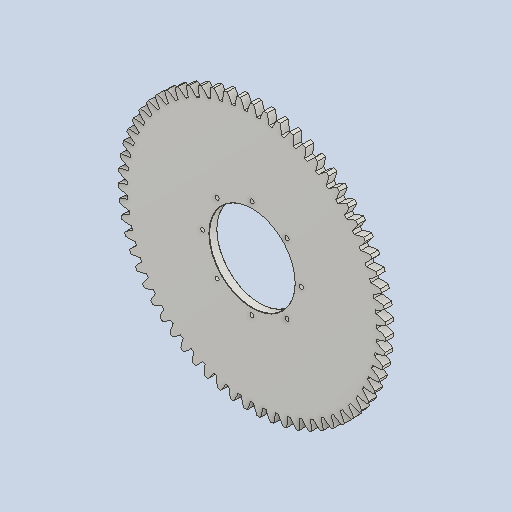
# Autodesk Inventor part: ДМФ 01 41 Шестерня ведомая
Saved by Autodesk Inventor 2024.2 (Build 282272000, 272)
## iProperties
CustomPartVersion: 1
Created: 2024-04-25
Part Number: ДМФ 01 41 Шестерня ведомая
Material: Steel
Document SubType Name: Modeling
Designer: pokla
Categories: <?xml version="1.0" encoding="UTF-16"?> <MemberInstance><Categories><FamilyTemplate><FamilyTemplateParameter ValueType="xs:double" Id="1" ObjectReferenceKey="da_z" ObjectType="kUserParameterObject"/><FamilyTemplateParameter ValueType="xs:double" Id="2" ObjectReferenceKey="da_b" ObjectType="kUserParameterObject"/><FamilyTemplateParameter ValueType="xs:double" Id="3" ObjectReferenceKey="da_beta" ObjectType="kUserParameterObject"/><FamilyTemplateParameter ValueType="xs:double" Id="4" ObjectReferenceKey="da_da" ObjectType="kUserParameterObject"/><FamilyTemplateParameter ValueType="xs:double" Id="5" ObjectReferenceKey="da_aw" ObjectType="kUserParameterObject"/><FamilyTemplateParameter ValueType="xs:string" Id="6" ObjectReferenceKey="EAIAABAAAACIAQAAAAAAAIAAAAAAAAAA" ObjectType="83910656" SubObjectId="SurfaceGeometry"/></FamilyTemplate><ParamToTemplateMap><ParamToTemplate CategoryParameter="//CategoryParameter[@InternalName='046C89C9-8512-4d59-83FE-43B91F4F132A']" TemplateParameter="1"/><ParamToTemplate CategoryParameter="//CategoryParameter[@InternalName='2552DF32-E462-4b46-AEBF-C6C7768E72AC']" TemplateParameter="2"/><ParamToTemplate CategoryParameter="//CategoryParameter[@InternalName='C9EE641D-15FC-4fae-A226-E94C4372FDD7']" TemplateParameter="3"/><ParamToTemplate><ParamToTemplate CategoryParameter="//CategoryParameter[@InternalName='00B6519A-459B-49c7-AD84-2E56D39A5744']" ConstantValue="0.000029"/></ParamToTemplate><ParamToTemplate><ParamToTemplate CategoryParameter="//CategoryParameter[@InternalName='04B31F0E-C7A6-4894-AA32-9629BEFACF47']" ConstantValue="1.000000"/></ParamToTemplate><ParamToTemplate><ParamToTemplate CategoryParameter="//CategoryParameter[@InternalName='43CBEC2E-7847-49e7-A936-2F7889FCB2D9']" ConstantValue="0.250000"/></ParamToTemplate><ParamToTemplate><ParamToTemplate CategoryParameter="//CategoryParameter[@InternalName='B1EFC894-105D-4ebd-86BF-FA20ED196853']" ConstantValue="0.333500"/></ParamToTemplate><ParamToTemplate><ParamToTemplate CategoryParameter="//CategoryParameter[@InternalName='51175063-3D10-4879-93E8-6246FE8B403D']" ConstantValue="2060000000.000000"/></ParamToTemplate><ParamToTemplate><ParamToTemplate CategoryParameter="//CategoryParameter[@InternalName='A3A52E27-4454-46a9-B0BD-C932399B70AF']" ConstantValue="0.300000"/></ParamToTemplate><ParamToTemplate><ParamToTemplate CategoryParameter="//CategoryParameter[@InternalName='91B76062-C214-41d9-B1B9-14D2AB99603D']" ConstantValue="1.250632"/></ParamToTemplate><ParamToTemplate><ParamToTemplate CategoryParameter="//CategoryParameter[@InternalName='374E806E-8B8A-4dda-A9AA-1039D6500AD2']" ConstantValue="0.799596"/></ParamToTemplate><ParamToTemplate><ParamToTemplate CategoryParameter="//CategoryParameter[@InternalName='2D373A89-B862-43d6-8D0B-0CBF12AB9F6C']" ConstantValue="0.253073"/></ParamToTemplate><ParamToTemplate CategoryParameter="//CategoryParameter[@InternalName='37777632-D6A2-4fac-9D53-DB8ACD95C989']" TemplateParameter="4"/><ParamToTemplate CategoryParameter="//CategoryParameter[@InternalName='FD1017F1-B727-4f7e-9707-0F86F1FF9423']" TemplateParameter="5"/><ParamToTemplate><ParamToTemplate CategoryParameter="//CategoryParameter[@InternalName='9E1B4470-B2D3-4ff1-B813-535BB4CDF51A']" ConstantValue="3520000.000000"/></ParamToTemplate><ParamToTemplate><ParamToTemplate CategoryParameter="//CategoryParameter[@InternalName='F8452263-BFF6-458c-9FB1-07C4B99E95CD']" ConstantValue="11400000.000000"/></ParamToTemplate><ParamToTemplate><ParamToTemplate CategoryParameter="//CategoryParameter[@InternalName='3E3BB259-FD49-497f-8171-6EBC954A3479']" ConstantValue="2.000000"/></ParamToTemplate><ParamToTemplate CategoryParameter="//CategoryParameter[@InternalName='27C3BAF2-7550-4e4b-AE2C-0DB134B7D9B7']" TemplateParameter="6"/></ParamToTemplateMap><Category DisplayName="Gear" InternalName="DC85795E-93AB-48d5-8EEE-5A27447B64BD" Mnemonic="Gear"><CategoryParameter DisplayName="z" InternalName="046C89C9-8512-4d59-83FE-43B91F4F132A" Mnemonic="z"/><CategoryParameter DisplayName="b" InternalName="2552DF32-E462-4b46-AEBF-C6C7768E72AC" Mnemonic="b"/><CategoryParameter DisplayName="||b|" InternalName="C9EE641D-15FC-4fae-A226-E94C4372FDD7" Mnemonic="beta"/><CategoryParameter DisplayName="x" InternalName="00B6519A-459B-49c7-AD84-2E56D39A5744" Mnemonic="x"/><CategoryParameter DisplayName="a*" InternalName="04B31F0E-C7A6-4894-AA32-9629BEFACF47" Mnemonic="a"/><CategoryParameter DisplayName="c*" InternalName="43CBEC2E-7847-49e7-A936-2F7889FCB2D9" Mnemonic="c"/><CategoryParameter DisplayName="r|.f|*" InternalName="B1EFC894-105D-4ebd-86BF-FA20ED196853" Mnemonic="rf"/><CategoryParameter DisplayName="E" InternalName="51175063-3D10-4879-93E8-6246FE8B403D" Mnemonic="E"/><CategoryParameter DisplayName="||m|" InternalName="A3A52E27-4454-46a9-B0BD-C932399B70AF" Mnemonic="mi"/><Category DisplayName="SpurGear" InternalName="26C5A22E-A91E-4dfd-A3B3-23CCAFAE1764" Mnemonic="SpurGear"><CategoryParameter DisplayName="m" InternalName="91B76062-C214-41d9-B1B9-14D2AB99603D" Mnemonic="m"/><CategoryParameter DisplayName="P" InternalName="374E806E-8B8A-4dda-A9AA-1039D6500AD2" Mnemonic="PP"/><CategoryParameter DisplayName="||a|" InternalName="2D373A89-B862-43d6-8D0B-0CBF12AB9F6C" Mnemonic="alpha"/><CategoryParameter DisplayName="d|.a|" InternalName="37777632-D6A2-4fac-9D53-DB8ACD95C989" Mnemonic="da"/><CategoryParameter DisplayName="a|.w|" InternalName="FD1017F1-B727-4f7e-9707-0F86F1FF9423" Mnemonic="aw"/><CategoryParameter DisplayName="||s||.Flim|" InternalName="9E1B4470-B2D3-4ff1-B813-535BB4CDF51A" Mnemonic="sFlim"/><CategoryParameter DisplayName="||s||.Hlim|" InternalName="F8452263-BFF6-458c-9FB1-07C4B99E95CD" Mnemonic="sHlim"/><CategoryParameter DisplayName="type" InternalName="3E3BB259-FD49-497f-8171-6EBC954A3479" Mnemonic="type"/><CategoryParameter DisplayName="PitchDiameter" InternalName="27C3BAF2-7550-4e4b-AE2C-0DB134B7D9B7" Mnemonic="IDS_PITCHDIAM"/></Category></Category></Categories></MemberInstance>
Density: 1 g/cm^3
Appearance: Steel
Author: pokla
Autodesk Inventor part; units mm, degrees
ref_plane "YZ Plane" through (0, 0, 0) normal (1, 0, 0) x (0, 1, 0)
ref_plane "XZ Plane" through (0, 0, 0) normal (0, 1, 0) x (-1, 0, 0)
ref_plane "XY Plane" through (0, 0, 0) normal (0, 0, 1) x (1, 0, 0)
sketch "Sketch1" plane through (0, 0, 0) normal (0, 0, 1) x (1, 0, 0)
  circle A0 centre (0, 0) radius 406.4558
  dimension "d0" = 812.9115
  constraints: 1 centre point
  measures "d0" diameter of A0
extrude "Extrusion1" add sketch "Sketch1" along normal blind 24
ref_plane "Work Plane2" through (0, 0, 12) normal (0, 0, 1) x (1, 0, 0)
sketch "Sketch2" plane through (0, 0, 0) normal (0, 0, -1) x (-1, 0, 0)
  circle A0 centre (0, 0) radius 406.4558 projected
  circle A1 centre (0, 0) radius 393.9491
  dimension "d3" = 787.8982
  constraints: 1 centre point, 1 coincident
  measures "d3" diameter of A1
surface extrude "Pitch Diameter" sketch "Sketch2" against normal through all shown no curves A1
ref_plane "Work Plane8" through (0, 0, 0) normal (0.9987569, 0.0498459, 0) x (0, 0, 1)
ref_plane "Work Plane9" through (0, 0, 0) normal (1, 0, 0) x (0, 1, 0)
spur gear teeth "Spur Gear" teeth 63 pitch diameter 787.8982 tip diameter 812.9115 root diameter 756.6331 face width 24 start plane through (0, 0, 0) normal (0, 0, -1) x (-1, 0, 0)
sketch "Sketch3" plane through (0, 0, 24) normal (0, 0, 1) x (1, 0, 0)
  arc A0 (-35.425, 404.9091) -> (-45.5086, 403.9001) centre (0, 0) ccw projected
  arc A1 (-45.5086, 403.9001) -> (-51.7172, 374.7649) centre (107.0022, 356.1713) ccw projected
  arc A2 (-51.7172, 374.7649) -> (-61.0443, 373.3591) centre (0, 0) ccw projected
  arc A3 (-61.0443, 373.3591) -> (-75.5648, 399.3698) centre (-207.2317, 308.8081) ccw projected
  arc A4 (-75.5648, 399.3698) -> (-85.4979, 397.3618) centre (0, 0) ccw projected
  arc A5 (-85.4979, 397.3618) -> (-88.7748, 367.7532) centre (71.0072, 365.0554) ccw projected
  arc A6 (-88.7748, 367.7532) -> (-97.9155, 365.4257) centre (0, 0) ccw projected
  arc A7 (-97.9155, 365.4257) -> (-114.9537, 389.8614) centre (-236.9493, 286.64) ccw projected
  arc A8 (-114.9537, 389.8614) -> (-124.6375, 386.8744) centre (0, 0) ccw projected
  arc A9 (-124.6375, 386.8744) -> (-124.95, 357.0867) centre (34.3066, 370.3114) ccw projected
  arc A10 (-124.95, 357.0867) -> (-133.8136, 353.8606) centre (0, 0) ccw projected
  arc A11 (-133.8136, 353.8606) -> (-153.2002, 376.4784) centre (-264.3119, 261.6231) ccw projected
  arc A12 (-153.2002, 376.4784) -> (-162.5384, 372.542) centre (0, 0) ccw projected
  arc A13 (-162.5384, 372.542) -> (-159.8835, 342.8712) centre (-2.735, 371.887) ccw projected
  arc A14 (-159.8835, 342.8712) -> (-168.3818, 338.7786) centre (0, 0) ccw projected
  arc A15 (-168.3818, 338.7786) -> (-189.924, 359.3538) centre (-289.0478, 234.0061) ccw projected
  arc A16 (-189.924, 359.3538) -> (-198.8239, 354.5072) centre (0, 0) ccw projected
  arc A17 (-198.8239, 354.5072) -> (-193.2279, 325.2482) centre (-39.7494, 369.7667) ccw projected
  arc A18 (-193.2279, 325.2482) -> (-201.2765, 320.3298) centre (0, 0) ccw projected
  arc A19 (-201.2765, 320.3298) -> (-224.7603, 338.6578) centre (-310.9109, 204.0634) ccw projected
  arc A20 (-224.7603, 338.6578) -> (-233.1334, 332.9491) centre (0, 0) ccw projected
  arc A21 (-233.1334, 332.9491) -> (-224.652, 304.3926) centre (-76.3687, 363.9715) ccw projected
  arc A22 (-224.652, 304.3926) -> (-232.1709, 298.6973) centre (0, 0) ccw projected
  arc A23 (-232.1709, 298.6973) -> (-257.3629, 314.596) centre (-329.6841, 172.0926) ccw projected
  arc A24 (-257.3629, 314.596) -> (-265.126, 308.082) centre (0, 0) ccw projected
  arc A25 (-265.126, 308.082) -> (-253.8434, 280.5119) centre (-112.2291, 354.559) ccw projected
  arc A26 (-253.8434, 280.5119) -> (-260.7578, 274.0963) centre (0, 0) ccw projected
  arc A27 (-260.7578, 274.0963) -> (-287.4076, 287.4076) centre (-345.1807, 138.4115) ccw projected
  arc A28 (-287.4076, 287.4076) -> (-294.4836, 280.153) centre (0, 0) ccw projected
  arc A29 (-294.4836, 280.153) -> (-280.5119, 253.8434) centre (-146.9741, 341.6227) ccw projected
  arc A30 (-280.5119, 253.8434) -> (-286.7532, 246.7711) centre (0, 0) ccw projected
  arc A31 (-286.7532, 246.7711) -> (-314.596, 257.3629) centre (-357.2467, 103.3548) ccw projected
  arc A32 (-314.596, 257.3629) -> (-320.9144, 249.4398) centre (0, 0) ccw projected
  arc A33 (-320.9144, 249.4398) -> (-304.3926, 224.652) centre (-180.2584, 325.2912) ccw projected
  arc A34 (-304.3926, 224.652) -> (-309.8988, 216.9935) centre (0, 0) ccw projected
  arc A35 (-309.8988, 216.9935) -> (-338.6578, 224.7603) centre (-365.7623, 67.2709) ccw projected
  arc A36 (-338.6578, 224.7603) -> (-344.1559, 216.2475) centre (0, 0) ccw projected
  arc A37 (-344.1559, 216.2475) -> (-325.2482, 193.2279) centre (-211.7512, 305.7268) ccw projected
  arc A38 (-325.2482, 193.2279) -> (-329.9644, 185.0592) centre (0, 0) ccw projected
  arc A39 (-329.9644, 185.0592) -> (-359.3538, 189.924) centre (-370.6428, 30.5185) ccw projected
  arc A40 (-359.3538, 189.924) -> (-363.977, 180.9061) centre (0, 0) ccw projected
  arc A41 (-363.977, 180.9061) -> (-342.8712, 159.8835) centre (-241.1395, 283.124) ccw projected
  arc A42 (-342.8712, 159.8835) -> (-346.7507, 151.2858) centre (0, 0) ccw projected
  arc A43 (-346.7507, 151.2858) -> (-376.4784, 153.2002) centre (-371.8396, -6.5373) ccw projected
  arc A44 (-376.4784, 153.2002) -> (-380.1808, 143.7667) centre (0, 0) ccw projected
  arc A45 (-380.1808, 143.7667) -> (-357.0867, 124.95) centre (-268.1313, 257.7073) ccw projected
  arc A46 (-357.0867, 124.95) -> (-360.0908, 116.0088) centre (0, 0) ccw projected
  arc A47 (-360.0908, 116.0088) -> (-389.8614, 114.9537) centre (-369.341, -43.5281) ccw projected
  arc A48 (-389.8614, 114.9537) -> (-392.6061, 105.1985) centre (0, 0) ccw projected
  arc A49 (-392.6061, 105.1985) -> (-367.7532, 88.7748) centre (-292.4582, 229.7295) ccw projected
  arc A50 (-367.7532, 88.7748) -> (-369.8521, 79.5788) centre (0, 0) ccw projected
  arc A51 (-369.8521, 79.5788) -> (-399.3698, 75.5648) centre (-363.1716, -80.0863) ccw projected
  arc A52 (-399.3698, 75.5648) -> (-401.1296, 65.5848) centre (0, 0) ccw projected
  arc A53 (-401.1296, 65.5848) -> (-374.7649, 51.7172) centre (-313.8786, 199.4685) ccw projected
  arc A54 (-374.7649, 51.7172) -> (-375.9378, 42.358) centre (0, 0) ccw projected
  arc A55 (-375.9378, 42.358) -> (-404.9091, 35.425) centre (-353.3929, -115.8485) ccw projected
  arc A56 (-404.9091, 35.425) -> (-405.6664, 25.3193) centre (0, 0) ccw projected
  arc A57 (-405.6664, 25.3193) -> (-378.052, 14.1457) centre (-332.1795, 167.2251) ccw projected
  arc A58 (-378.052, 14.1457) -> (-378.2871, 4.7162) centre (0, 0) ccw projected
  arc A59 (-378.2871, 4.7162) -> (-406.4242, -5.067) centre (-340.1021, -150.4594) ccw projected
  arc A60 (-406.4242, -5.067) -> (-406.1715, -15.1979) centre (0, 0) ccw projected
  arc A61 (-406.1715, -15.1979) -> (-377.5818, -23.5664) centre (-347.1791, 133.3197) ccw projected
  arc A62 (-377.5818, -23.5664) -> (-376.8769, -32.9725) centre (0, 0) ccw projected
  arc A63 (-376.8769, -32.9725) -> (-403.9001, -45.5086) centre (-323.4311, -183.575) ccw projected
  arc A64 (-403.9001, -45.5086) -> (-402.64, -55.564) centre (0, 0) ccw projected
  arc A65 (-402.64, -55.564) -> (-373.3591, -61.0443) centre (-358.7282, 98.0893) ccw projected
  arc A66 (-373.3591, -61.0443) -> (-371.7211, -70.3334) centre (0, 0) ccw projected
  arc A67 (-371.7211, -70.3334) -> (-397.3618, -85.4979) centre (-303.5457, -214.8661) ccw projected
  arc A68 (-397.3618, -85.4979) -> (-395.1068, -95.3779) centre (0, 0) ccw projected
  arc A69 (-395.1068, -95.3779) -> (-365.4257, -97.9155) centre (-366.7122, 61.8841) ccw projected
  arc A70 (-365.4257, -97.9155) -> (-362.871, -106.9954) centre (0, 0) ccw projected
  arc A71 (-362.871, -106.9954) -> (-386.8744, -124.6375) centre (-280.6436, -244.0218) ccw projected
  arc A72 (-386.8744, -124.6375) -> (-383.6468, -134.2438) centre (0, 0) ccw projected
  arc A73 (-383.6468, -134.2438) -> (-353.8606, -133.8136) centre (-371.0515, 25.0638) ccw projected
  arc A74 (-353.8606, -133.8136) -> (-350.4145, -142.594) centre (0, 0) ccw projected
  arc A75 (-350.4145, -142.594) -> (-372.542, -162.5384) centre (-254.9523, -270.7522) ccw projected
  arc A76 (-372.542, -162.5384) -> (-368.374, -171.7756) centre (0, 0) ccw projected
  arc A77 (-368.374, -171.7756) -> (-338.7786, -168.3818) centre (-371.7033, -12.0055) ccw projected
  arc A78 (-338.7786, -168.3818) -> (-334.4755, -176.7755) centre (0, 0) ccw projected
  arc A79 (-334.4755, -176.7755) -> (-354.5072, -198.8239) centre (-226.7272, -294.7919) ccw projected
  arc A80 (-354.5072, -198.8239) -> (-349.4402, -207.6002) centre (0, 0) ccw projected
  arc A81 (-349.4402, -207.6002) -> (-320.3298, -201.2765) centre (-368.6608, -48.9556) ccw projected
  arc A82 (-320.3298, -201.2765) -> (-315.2122, -209.2) centre (0, 0) ccw projected
  arc A83 (-315.2122, -209.2) -> (-332.9491, -233.1334) centre (-196.2487, -315.9017) ccw projected
  arc A84 (-332.9491, -233.1334) -> (-327.0334, -241.3616) centre (0, 0) ccw projected
  arc A85 (-327.0334, -241.3616) -> (-298.6973, -232.1709) centre (-361.9545, -85.419) ccw projected
  arc A86 (-298.6973, -232.1709) -> (-292.8163, -239.5455) centre (0, 0) ccw projected
  arc A87 (-292.8163, -239.5455) -> (-308.082, -265.126) centre (-163.8199, -333.872) ccw projected
  arc A88 (-308.082, -265.126) -> (-301.3764, -272.7243) centre (0, 0) ccw projected
  arc A89 (-301.3764, -272.7243) -> (-274.0963, -260.7578) centre (-351.6508, -121.0336) ccw projected
  arc A90 (-274.0963, -260.7578) -> (-267.5102, -267.5102) centre (0, 0) ccw projected
  arc A91 (-267.5102, -267.5102) -> (-280.153, -294.4836) centre (-129.7629, -348.5241) ccw projected
  arc A92 (-280.153, -294.4836) -> (-272.7243, -301.3764) centre (0, 0) ccw projected
  arc A93 (-272.7243, -301.3764) -> (-246.7711, -286.7532) centre (-337.8523, -155.4453) ccw projected
  arc A94 (-246.7711, -286.7532) -> (-239.5455, -292.8163) centre (0, 0) ccw projected
  arc A95 (-239.5455, -292.8163) -> (-249.4398, -320.9144) centre (-94.4163, -359.7124) ccw projected
  arc A96 (-249.4398, -320.9144) -> (-241.3616, -327.0334) centre (0, 0) ccw projected
  arc A97 (-241.3616, -327.0334) -> (-216.9935, -309.8988) centre (-320.6961, -188.3121) ccw projected
  arc A98 (-216.9935, -309.8988) -> (-209.2, -315.2122) centre (0, 0) ccw projected
  arc A99 (-209.2, -315.2122) -> (-216.2475, -344.1559) centre (-58.1313, -367.3257) ccw projected
  arc A100 (-216.2475, -344.1559) -> (-207.6002, -349.4402) centre (0, 0) ccw projected
  arc A101 (-207.6002, -349.4402) -> (-185.0592, -329.9644) centre (-300.3527, -219.3073) ccw projected
  arc A102 (-185.0592, -329.9644) -> (-176.7755, -334.4755) centre (0, 0) ccw projected
  arc A103 (-176.7755, -334.4755) -> (-180.9061, -363.977) centre (-21.2686, -371.2884) ccw projected
  arc A104 (-180.9061, -363.977) -> (-171.7756, -368.374) centre (0, 0) ccw projected
  arc A105 (-171.7756, -368.374) -> (-151.2858, -346.7507) centre (-277.0242, -248.123) ccw projected
  arc A106 (-151.2858, -346.7507) -> (-142.594, -350.4145) centre (0, 0) ccw projected
  arc A107 (-142.594, -350.4145) -> (-143.7667, -380.1808) centre (15.8055, -371.5611) ccw projected
  arc A108 (-143.7667, -380.1808) -> (-134.2438, -383.6468) centre (0, 0) ccw projected
  arc A109 (-134.2438, -383.6468) -> (-116.0088, -360.0908) centre (-250.9425, -274.4727) ccw projected
  arc A110 (-116.0088, -360.0908) -> (-106.9954, -362.871) centre (0, 0) ccw projected
  arc A111 (-106.9954, -362.871) -> (-105.1985, -392.6061) centre (52.7225, -368.141) ccw projected
  arc A112 (-105.1985, -392.6061) -> (-95.3779, -395.1068) centre (0, 0) ccw projected
  arc A113 (-95.3779, -395.1068) -> (-79.5788, -369.8521) centre (-222.3669, -298.0946) ccw projected
  arc A114 (-79.5788, -369.8521) -> (-70.3334, -371.7211) centre (0, 0) ccw projected
  arc A115 (-70.3334, -371.7211) -> (-65.5848, -401.1296) centre (89.1155, -361.0621) ccw projected
  arc A116 (-65.5848, -401.1296) -> (-55.564, -402.64) centre (0, 0) ccw projected
  arc A117 (-55.564, -402.64) -> (-42.358, -375.9378) centre (-191.5813, -318.7539) ccw projected
  arc A118 (-42.358, -375.9378) -> (-32.9725, -376.8769) centre (0, 0) ccw projected
  arc A119 (-32.9725, -376.8769) -> (-25.3193, -405.6664) centre (124.6228, -350.3949) ccw projected
  arc A120 (-25.3193, -405.6664) -> (-15.1979, -406.1715) centre (0, 0) ccw projected
  arc A121 (-15.1979, -406.1715) -> (-4.7162, -378.2871) centre (-158.8916, -336.2453) ccw projected
  arc A122 (-4.7162, -378.2871) -> (4.7162, -378.2871) centre (0, 0) ccw projected
  arc A123 (4.7162, -378.2871) -> (15.1979, -406.1715) centre (158.8916, -336.2453) ccw projected
  arc A124 (15.1979, -406.1715) -> (25.3193, -405.6664) centre (0, 0) ccw projected
  arc A125 (25.3193, -405.6664) -> (32.9725, -376.8769) centre (-124.6228, -350.3949) ccw projected
  arc A126 (32.9725, -376.8769) -> (42.358, -375.9378) centre (0, 0) ccw projected
  arc A127 (42.358, -375.9378) -> (55.564, -402.64) centre (191.5813, -318.7539) ccw projected
  arc A128 (55.564, -402.64) -> (65.5848, -401.1296) centre (0, 0) ccw projected
  arc A129 (65.5848, -401.1296) -> (70.3334, -371.7211) centre (-89.1155, -361.0621) ccw projected
  arc A130 (70.3334, -371.7211) -> (79.5788, -369.8521) centre (0, 0) ccw projected
  arc A131 (79.5788, -369.8521) -> (95.3779, -395.1068) centre (222.3669, -298.0946) ccw projected
  arc A132 (95.3779, -395.1068) -> (105.1985, -392.6061) centre (0, 0) ccw projected
  arc A133 (105.1985, -392.6061) -> (106.9954, -362.871) centre (-52.7225, -368.141) ccw projected
  arc A134 (106.9954, -362.871) -> (116.0088, -360.0908) centre (0, 0) ccw projected
  arc A135 (116.0088, -360.0908) -> (134.2438, -383.6468) centre (250.9425, -274.4727) ccw projected
  arc A136 (134.2438, -383.6468) -> (143.7667, -380.1808) centre (0, 0) ccw projected
  arc A137 (143.7667, -380.1808) -> (142.594, -350.4145) centre (-15.8055, -371.5611) ccw projected
  arc A138 (142.594, -350.4145) -> (151.2858, -346.7507) centre (0, 0) ccw projected
  arc A139 (151.2858, -346.7507) -> (171.7756, -368.374) centre (277.0242, -248.123) ccw projected
  arc A140 (171.7756, -368.374) -> (180.9061, -363.977) centre (0, 0) ccw projected
  arc A141 (180.9061, -363.977) -> (176.7755, -334.4755) centre (21.2686, -371.2884) ccw projected
  arc A142 (176.7755, -334.4755) -> (185.0592, -329.9644) centre (0, 0) ccw projected
  arc A143 (185.0592, -329.9644) -> (207.6002, -349.4402) centre (300.3527, -219.3073) ccw projected
  arc A144 (207.6002, -349.4402) -> (216.2475, -344.1559) centre (0, 0) ccw projected
  arc A145 (216.2475, -344.1559) -> (209.2, -315.2122) centre (58.1313, -367.3257) ccw projected
  arc A146 (209.2, -315.2122) -> (216.9935, -309.8988) centre (0, 0) ccw projected
  arc A147 (216.9935, -309.8988) -> (241.3616, -327.0334) centre (320.6961, -188.3121) ccw projected
  arc A148 (241.3616, -327.0334) -> (249.4398, -320.9144) centre (0, 0) ccw projected
  arc A149 (249.4398, -320.9144) -> (239.5455, -292.8163) centre (94.4163, -359.7124) ccw projected
  arc A150 (239.5455, -292.8163) -> (246.7711, -286.7532) centre (0, 0) ccw projected
  arc A151 (246.7711, -286.7532) -> (272.7243, -301.3764) centre (337.8523, -155.4453) ccw projected
  arc A152 (272.7243, -301.3764) -> (280.153, -294.4836) centre (0, 0) ccw projected
  arc A153 (280.153, -294.4836) -> (267.5102, -267.5102) centre (129.7629, -348.5241) ccw projected
  arc A154 (267.5102, -267.5102) -> (274.0963, -260.7578) centre (0, 0) ccw projected
  arc A155 (274.0963, -260.7578) -> (301.3764, -272.7243) centre (351.6508, -121.0336) ccw projected
  arc A156 (301.3764, -272.7243) -> (308.082, -265.126) centre (0, 0) ccw projected
  arc A157 (308.082, -265.126) -> (292.8163, -239.5455) centre (163.8199, -333.872) ccw projected
  arc A158 (292.8163, -239.5455) -> (298.6973, -232.1709) centre (0, 0) ccw projected
  arc A159 (298.6973, -232.1709) -> (327.0334, -241.3616) centre (361.9545, -85.419) ccw projected
  arc A160 (327.0334, -241.3616) -> (332.9491, -233.1334) centre (0, 0) ccw projected
  arc A161 (332.9491, -233.1334) -> (315.2122, -209.2) centre (196.2487, -315.9017) ccw projected
  arc A162 (315.2122, -209.2) -> (320.3298, -201.2765) centre (0, 0) ccw projected
  arc A163 (320.3298, -201.2765) -> (349.4402, -207.6002) centre (368.6608, -48.9556) ccw projected
  arc A164 (349.4402, -207.6002) -> (354.5072, -198.8239) centre (0, 0) ccw projected
  arc A165 (354.5072, -198.8239) -> (334.4755, -176.7755) centre (226.7272, -294.7919) ccw projected
  arc A166 (334.4755, -176.7755) -> (338.7786, -168.3818) centre (0, 0) ccw projected
  arc A167 (338.7786, -168.3818) -> (368.374, -171.7756) centre (371.7033, -12.0055) ccw projected
  arc A168 (368.374, -171.7756) -> (372.542, -162.5384) centre (0, 0) ccw projected
  arc A169 (372.542, -162.5384) -> (350.4145, -142.594) centre (254.9523, -270.7522) ccw projected
  arc A170 (350.4145, -142.594) -> (353.8606, -133.8136) centre (0, 0) ccw projected
  arc A171 (353.8606, -133.8136) -> (383.6468, -134.2438) centre (371.0515, 25.0638) ccw projected
  arc A172 (383.6468, -134.2438) -> (386.8744, -124.6375) centre (0, 0) ccw projected
  arc A173 (386.8744, -124.6375) -> (362.871, -106.9954) centre (280.6436, -244.0218) ccw projected
  arc A174 (362.871, -106.9954) -> (365.4257, -97.9155) centre (0, 0) ccw projected
  arc A175 (365.4257, -97.9155) -> (395.1068, -95.3779) centre (366.7122, 61.8841) ccw projected
  arc A176 (395.1068, -95.3779) -> (397.3618, -85.4979) centre (0, 0) ccw projected
  arc A177 (397.3618, -85.4979) -> (371.7211, -70.3334) centre (303.5457, -214.8661) ccw projected
  arc A178 (371.7211, -70.3334) -> (373.3591, -61.0443) centre (0, 0) ccw projected
  arc A179 (373.3591, -61.0443) -> (402.64, -55.564) centre (358.7282, 98.0893) ccw projected
  arc A180 (402.64, -55.564) -> (403.9001, -45.5086) centre (0, 0) ccw projected
  arc A181 (403.9001, -45.5086) -> (376.8769, -32.9725) centre (323.4311, -183.575) ccw projected
  arc A182 (376.8769, -32.9725) -> (377.5818, -23.5664) centre (0, 0) ccw projected
  arc A183 (377.5818, -23.5664) -> (406.1715, -15.1979) centre (347.1791, 133.3197) ccw projected
  arc A184 (406.1715, -15.1979) -> (406.4242, -5.067) centre (0, 0) ccw projected
  arc A185 (406.4242, -5.067) -> (378.2871, 4.7162) centre (340.1021, -150.4594) ccw projected
  arc A186 (378.2871, 4.7162) -> (378.052, 14.1457) centre (0, 0) ccw projected
  arc A187 (378.052, 14.1457) -> (405.6664, 25.3193) centre (332.1795, 167.2251) ccw projected
  arc A188 (405.6664, 25.3193) -> (404.9091, 35.425) centre (0, 0) ccw projected
  arc A189 (404.9091, 35.425) -> (375.9378, 42.358) centre (353.3929, -115.8485) ccw projected
  arc A190 (375.9378, 42.358) -> (374.7649, 51.7172) centre (0, 0) ccw projected
  arc A191 (374.7649, 51.7172) -> (401.1296, 65.5848) centre (313.8786, 199.4685) ccw projected
  arc A192 (401.1296, 65.5848) -> (399.3698, 75.5648) centre (0, 0) ccw projected
  arc A193 (399.3698, 75.5648) -> (369.8521, 79.5788) centre (363.1716, -80.0863) ccw projected
  arc A194 (369.8521, 79.5788) -> (367.7532, 88.7748) centre (0, 0) ccw projected
  arc A195 (367.7532, 88.7748) -> (392.6061, 105.1985) centre (292.4582, 229.7295) ccw projected
  arc A196 (392.6061, 105.1985) -> (389.8614, 114.9537) centre (0, 0) ccw projected
  arc A197 (389.8614, 114.9537) -> (360.0908, 116.0088) centre (369.341, -43.5281) ccw projected
  arc A198 (360.0908, 116.0088) -> (357.0867, 124.95) centre (0, 0) ccw projected
  arc A199 (357.0867, 124.95) -> (380.1808, 143.7667) centre (268.1313, 257.7073) ccw projected
  arc A200 (380.1808, 143.7667) -> (376.4784, 153.2002) centre (0, 0) ccw projected
  arc A201 (376.4784, 153.2002) -> (346.7507, 151.2858) centre (371.8396, -6.5373) ccw projected
  arc A202 (346.7507, 151.2858) -> (342.8712, 159.8835) centre (0, 0) ccw projected
  arc A203 (342.8712, 159.8835) -> (363.977, 180.9061) centre (241.1395, 283.124) ccw projected
  arc A204 (363.977, 180.9061) -> (359.3538, 189.924) centre (0, 0) ccw projected
  arc A205 (359.3538, 189.924) -> (329.9644, 185.0592) centre (370.6428, 30.5185) ccw projected
  arc A206 (329.9644, 185.0592) -> (325.2482, 193.2279) centre (0, 0) ccw projected
  arc A207 (325.2482, 193.2279) -> (344.1559, 216.2475) centre (211.7512, 305.7268) ccw projected
  arc A208 (344.1559, 216.2475) -> (338.6578, 224.7603) centre (0, 0) ccw projected
  arc A209 (338.6578, 224.7603) -> (309.8988, 216.9935) centre (365.7623, 67.2709) ccw projected
  arc A210 (309.8988, 216.9935) -> (304.3926, 224.652) centre (0, 0) ccw projected
  arc A211 (304.3926, 224.652) -> (320.9144, 249.4398) centre (180.2584, 325.2912) ccw projected
  arc A212 (320.9144, 249.4398) -> (314.596, 257.3629) centre (0, 0) ccw projected
  arc A213 (314.596, 257.3629) -> (286.7532, 246.7711) centre (357.2467, 103.3548) ccw projected
  arc A214 (286.7532, 246.7711) -> (280.5119, 253.8434) centre (0, 0) ccw projected
  arc A215 (280.5119, 253.8434) -> (294.4836, 280.153) centre (146.9741, 341.6227) ccw projected
  arc A216 (294.4836, 280.153) -> (287.4076, 287.4076) centre (0, 0) ccw projected
  arc A217 (287.4076, 287.4076) -> (260.7578, 274.0963) centre (345.1807, 138.4115) ccw projected
  arc A218 (260.7578, 274.0963) -> (253.8434, 280.5119) centre (0, 0) ccw projected
  arc A219 (253.8434, 280.5119) -> (265.126, 308.082) centre (112.2291, 354.559) ccw projected
  arc A220 (265.126, 308.082) -> (257.3629, 314.596) centre (0, 0) ccw projected
  arc A221 (257.3629, 314.596) -> (232.1709, 298.6973) centre (329.6841, 172.0926) ccw projected
  arc A222 (232.1709, 298.6973) -> (224.652, 304.3926) centre (0, 0) ccw projected
  arc A223 (224.652, 304.3926) -> (233.1334, 332.9491) centre (76.3687, 363.9715) ccw projected
  arc A224 (233.1334, 332.9491) -> (224.7603, 338.6578) centre (0, 0) ccw projected
  arc A225 (224.7603, 338.6578) -> (201.2765, 320.3298) centre (310.9109, 204.0634) ccw projected
  arc A226 (201.2765, 320.3298) -> (193.2279, 325.2482) centre (0, 0) ccw projected
  arc A227 (193.2279, 325.2482) -> (198.8239, 354.5072) centre (39.7494, 369.7667) ccw projected
  arc A228 (198.8239, 354.5072) -> (189.924, 359.3538) centre (0, 0) ccw projected
  arc A229 (189.924, 359.3538) -> (168.3818, 338.7786) centre (289.0478, 234.0061) ccw projected
  arc A230 (168.3818, 338.7786) -> (159.8835, 342.8712) centre (0, 0) ccw projected
  arc A231 (159.8835, 342.8712) -> (162.5384, 372.542) centre (2.735, 371.887) ccw projected
  arc A232 (162.5384, 372.542) -> (153.2002, 376.4784) centre (0, 0) ccw projected
  arc A233 (153.2002, 376.4784) -> (133.8136, 353.8606) centre (264.3119, 261.6231) ccw projected
  arc A234 (133.8136, 353.8606) -> (124.95, 357.0867) centre (0, 0) ccw projected
  arc A235 (124.95, 357.0867) -> (124.6375, 386.8744) centre (-34.3066, 370.3114) ccw projected
  arc A236 (124.6375, 386.8744) -> (114.9537, 389.8614) centre (0, 0) ccw projected
  arc A237 (114.9537, 389.8614) -> (97.9155, 365.4257) centre (236.9493, 286.64) ccw projected
  arc A238 (97.9155, 365.4257) -> (88.7748, 367.7532) centre (0, 0) ccw projected
  arc A239 (88.7748, 367.7532) -> (85.4979, 397.3618) centre (-71.0072, 365.0554) ccw projected
  arc A240 (85.4979, 397.3618) -> (75.5648, 399.3698) centre (0, 0) ccw projected
  arc A241 (75.5648, 399.3698) -> (61.0443, 373.3591) centre (207.2317, 308.8081) ccw projected
  arc A242 (61.0443, 373.3591) -> (51.7172, 374.7649) centre (0, 0) ccw projected
  arc A243 (51.7172, 374.7649) -> (45.5086, 403.9001) centre (-107.0022, 356.1713) ccw projected
  arc A244 (45.5086, 403.9001) -> (35.425, 404.9091) centre (0, 0) ccw projected
  arc A245 (35.425, 404.9091) -> (23.5664, 377.5818) centre (175.4545, 327.9072) ccw projected
  arc A246 (23.5664, 377.5818) -> (14.1457, 378.052) centre (0, 0) ccw projected
  arc A247 (14.1457, 378.052) -> (5.067, 406.4242) centre (-141.9337, 343.7474) ccw projected
  arc A248 (5.067, 406.4242) -> (-5.067, 406.4242) centre (0, 0) ccw projected
  arc A249 (-5.067, 406.4242) -> (-14.1457, 378.052) centre (141.9337, 343.7474) ccw projected
  arc A250 (-14.1457, 378.052) -> (-23.5664, 377.5818) centre (0, 0) ccw projected
  arc A251 (-23.5664, 377.5818) -> (-35.425, 404.9091) centre (-175.4545, 327.9072) ccw projected
  circle A252 centre (0, 0) radius 130
  dimension "d49" = 260
  constraints: 1 centre point, 1 concentric
  measures "d49" diameter of A252
extrude "Extrusion2" cut sketch "Sketch3" against normal through all contours A252
sketch "Sketch4" plane through (0, 0, 24) normal (0, 0, 1) x (1, 0, 0)
  circle A0 centre (0, 150) radius 6.25
  point P0 (0, 0)
  dimension "d52" = 12.5
  dimension "d53" = 150
  constraints: 1 centre point, 1 vertical alignment
  measures "d52" diameter of A0
  measures "d53" distance of point (0, 0) A0.centre
extrude "Extrusion3" cut sketch "Sketch4" against normal through all
pattern_circular "Circular Pattern1" count 8 over 360 about axis through (0, 0, 0) along (0, 0, 1) of "Extrusion3"
fillet "Fillet1" radius 1 2 edges at (-130, 0, 24) (-130, 0, 0)
equation "\"d0\" = da_da"
equation "\"d1\" = da_b"
equation "\"d49\" = Вал_ось_диаметр_НОС"
equation "\"d3\" = da_d"
equation "\"d16\" = da_aw"
equation "\"d43\" = da_aw"
equation "\"d46\" = da_aw"
equation "\"da_da\" = 812.91152"
equation "\"da_b\" = 24"
equation "\"Вал_ось_диаметр_НОС\" = 260"
equation "\"da_d\" = 787.89816"
equation "\"da_aw\" = 494"
body "Solid1"
body "Srf1"
